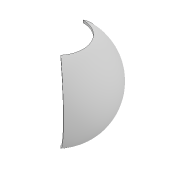
# Autodesk Inventor part: Sphere_cover
Saved by Autodesk Inventor 2022 (Build 260153000, 153)
## iProperties
Created: 2022-08-08
Part Number: Sphere_cover
Material: Generic
Document SubType Name: Modeling
Designer: dell
Density: 1 g/cm^3
Appearance: Default
Author: dell
Autodesk Inventor part; units mm, degrees
ref_plane "YZ Plane" through (0, 0, 0) normal (1, 0, 0) x (0, 1, 0)
ref_plane "XZ Plane" through (0, 0, 0) normal (0, 1, 0) x (-1, 0, 0)
ref_plane "XY Plane" through (0, 0, 0) normal (0, 0, 1) x (1, 0, 0)
sketch "Sketch2" plane through (0, 0, 0) normal (1, 0, 0) x (0, 1, 0)
  arc A0 (-45, 0) -> (45, 0) centre (0, 0) ccw
  arc A1 (-47, 0) -> (47, 0) centre (0, 0) ccw
  line L0 (-45, 0) -> (-47, 0)
  line L1 (45, 0) -> (47, 0)
  line L2 (-65.8, 0) -> (65.8, 0) projected
  line L3 (0, -56.4) -> (0, 9.4) projected
  dimension "d8" = 2
  dimension "d9" = 45
  constraints: 4 end point, 4 point on circle, 2 centre point, 2 collinear, 2 horizontal
  measures "d8" radial gap between concentric circles of A0 A1
  measures "d9" radius of A0
revolve "Revolution1" add sketch "Sketch2" angle 130 about axis through (0, -10, 0) along (0, -1, 0) contours A0 L3 A1 L0 | A0 L1 A1 L3
sketch "Sketch3" plane through (0, 0, 0) normal (0, 1, 0) x (-1, 0, 0)
  circle A0 centre (0, 0) radius 25
  dimension "d12" = 50
  constraints: 1 centre point, 1 coincident
  measures "d12" diameter of A0
extrude "Extrusion1" cut sketch "Sketch3" along normal mid plane 100
body "Solid1"
